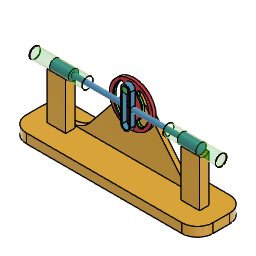
ScotchYoke (Autodesk Fusion 360 design; units mm, degrees)
Autodesk Fusion 360 part; units mm, degrees
sketch "BaseSketch" plane through (0, 0, 0) normal (0, 0, 1) x (1, 0, 0) in component "Holder"
  line L0 (30, 4.8) -> (30, 7.5)
  line L1 (27.5, 10) -> (2.5, 10)
  line L2 (0, 7.5) -> (0, 4.8)
  arc A0 (2.5, 10) -> (0, 7.5) centre (2.5, 7.5) ccw
  arc A1 (30, 7.5) -> (27.5, 10) centre (27.5, 7.5) ccw
  line L3 (15, 0) -> (15, 10) construction
  line L4 (2.75, 6.5) -> (2.75, 5.8)
  line L5 (5.75, 6.15) -> (5.75, 6.9)
  line L6 (5.75, 6.9) -> (2.75, 6.9)
  line L7 (2.75, 6.9) -> (2.75, 5.4)
  line L8 (2.75, 5.4) -> (5.75, 5.4)
  line L9 (5.75, 5.4) -> (5.75, 6.9)
  line L10 (5.75, 2.3) -> (2.5, 2.3)
  line L11 (0, 2.3) -> (0, 2.5)
  line L12 (5.75, 2.3) -> (27.5, 2.3)
  arc A2 (0, 4.8) -> (2.5, 2.3) centre (2.5, 4.8) ccw
  arc A3 (27.5, 2.3) -> (30, 4.8) centre (27.5, 4.8) ccw
  line L13 (27.25, 6.9) -> (27.25, 5.4)
  line L14 (24.25, 6.9) -> (27.25, 6.9)
  line L15 (24.25, 5.4) -> (24.25, 6.9)
  line L16 (27.25, 5.4) -> (24.25, 5.4)
  point P0 (30, 0)
  point P1 (0, 10)
  point P2 (27.5, 7.5)
  dimension "d1" = 30
  dimension "d3" = 2.5
  dimension "d4" = 2.5
  dimension "d81" = 3
  dimension "d82" = 1.5
  dimension "d83" = 3.1
  dimension "d84" = 2.5
  dimension "d85" = 2.5
  constraint vertical L0
  constraint horizontal L1
  constraint vertical L2
  constraint coincident P1 L1
  constraint coincident P1 L2
  constraint tangent L1 A0
  constraint tangent L2 A0
  constraint tangent L0 A1
  constraint tangent L1 A1
  constraint coincident P0 L0
  constraint coincident origin L2
  constraint midpoint L1 L3.end
  constraint vertical L4
  constraint horizontal L6
  constraint vertical L7
  constraint horizontal L8
  constraint vertical L9
  constraint perpendicular L10 L11
  constraint perpendicular L0 L12
  constraint coincident L11.start L10
  constraint coincident L2 L11.end
  constraint tangent L10 A2
  constraint tangent L2 A2
  constraint tangent L12 A3
  constraint tangent L0 A3
  constraint symmetric A0.centre L3 P2
  constraint symmetric L3 L5.end L14.start
  constraint symmetric L3 L6.end L13.start
  constraint symmetric L3 L7.end L13.end
  constraint symmetric L3 L8.end L15.start
  measures "d1" distance of origin P0
  measures "d3" radius of A0
  measures "d4" radius of A1
  measures "d81" distance of L5.end L6.end
  measures "d82" distance of L5.end L8.end
  measures "d83" distance of L8.end L10.start
  measures "d84" radius of A2
  measures "d85" radius of A3
extrude "Extrude1" add sketch "BaseSketch" along normal blind 1.5 contours L0 L1 L2 A0 A1 L10 L12 A2 A3 | L4 L5 L6 L7 L8 L9 | L13 L14 L15 L16 makes body 1 in component "Holder"
sketch "CrankSupportSketch" plane through (0, 0, 0) normal (0, 1, 0) x (1, 0, 0) in component "Holder"
  line L0 (13.2512, -9.8397) -> (6.5, -1.5)
  line L1 (6.5, -1.5) -> (15, -1.5)
  line L2 (16.7488, -9.8397) -> (23.5, -1.5)
  line L3 (23.5, -1.5) -> (15, -1.5)
  arc A0 (13.2512, -9.8397) -> (16.7488, -9.8397) centre (15, -8.424) ccw
  circle A1 centre (15, -9.5) radius 0.5
  line L4 (15, -9.5) -> (2.1474, -9.5)
  dimension "d12" = 2.25
  dimension "d13" = 1
  constraint horizontal L1
  constraint tangent L0 A0
  constraint tangent L2 A0
  constraint coincident A1.centre L4.start
  constraint horizontal L4
  measures "d12" radius of A0
  measures "d13" diameter of A1
extrude "Extrude3" add sketch "CrankSupportSketch" against normal blind 0.75 from surface at 8 contours L0 L1 L2 L3 A0 | A1 bodies 1 in component "Holder"
extrude "Extrude4" cut sketch "CrankSupportSketch" along normal blind 7.75 contours A1 bodies 1 in component "Holder"
move_face "OffsetFaces1" offset -0.05 1 faces at (15.3986, 7.4167, 9.1981) on bodies 1 in component "Holder"
fillet "Fillet1" radius 4.25 1 edges at (23.5, 7.625, 1.5) on bodies 1 in component "Holder"
fillet "Fillet2" radius 4.25 1 edges at (6.5, 7.625, 1.5) on bodies 1 in component "Holder"
sketch "CrankSketch" plane through (0, 7.75, 0) normal (0, -1, 0) x (1, 0, 0) in component "Crank"
  circle A0 centre (15, 9.5) radius 0.55
  circle A1 centre (15, 9.5) radius 3.5
  circle A2 centre (15, 9.5) radius 0.55
  circle A3 centre (15, 9.5) radius 0.5
  circle A4 centre (15, 12) radius 0.5
  line L0 (13.5, 7.5) -> (14, 7.5) construction
  line L1 (13.5, 11.5) -> (14, 11.5) construction
  arc A5 (13.8536, 11.1464) -> (13.1464, 11.8536) centre (13.5, 11.5) ccw
  arc A6 (13.1464, 7.1464) -> (13.8536, 7.8536) centre (13.5, 7.5) ccw
  arc A7 (13.1464, 11.8536) -> (13.1464, 7.1464) centre (15.5, 9.5) ccw
  arc A8 (13.8536, 11.1464) -> (13.8536, 7.8536) centre (15.5, 9.5) ccw
  arc A9 (16.1005, 7.8536) -> (16.1005, 11.1464) centre (14.454, 9.5) ccw
  arc A10 (16.8076, 11.8536) -> (16.1005, 11.1464) centre (16.454, 11.5) ccw
  arc A11 (16.8076, 7.1464) -> (16.8076, 11.8536) centre (14.454, 9.5) ccw
  arc A12 (16.1005, 7.8536) -> (16.8076, 7.1464) centre (16.454, 7.5) ccw
  dimension "d34" = 1
  constraint concentric A0 A1
  constraint concentric A0 A2
  constraint concentric A1 A3
  constraint horizontal L0
  constraint coincident L0.start A6.centre
  constraint horizontal L1
  constraint coincident L1.start A5.centre
  constraint tangent A6 A7
  constraint tangent A6 A8
  measures "d34" diameter of A3
extrude "Extrude1'" add sketch "CrankSketch" along normal blind 0.5 from surface at 0.6 separate body contours A0 A2 | A1 makes body 2 in component "Crank"
extrude "Extrude2" add sketch "CrankSketch" along normal blind 1.5 from surface at 0.6 contours A4 bodies 2 in component "Crank"
extrude "Extrude3'" add sketch "CrankSketch" along normal blind 1.2 from surface at 0.05 contours A3 bodies 2 in component "Crank"
sketch "SliderSketch" plane through (0, 6.65, 0) normal (0, -1, 0) x (1, 0, 0) in component "Slider&Piston"
  arc A0 (13.1464, 11.8536) -> (13.1464, 7.1464) centre (15.5, 9.5) ccw
  arc A1 (13.8536, 11.1464) -> (13.1464, 11.8536) centre (13.5, 11.5) ccw
  arc A2 (13.8536, 11.1464) -> (13.8536, 7.8536) centre (15.5, 9.5) ccw
  arc A3 (13.1464, 7.1464) -> (13.8536, 7.8536) centre (13.5, 7.5) ccw
  arc A4 (16.1005, 7.8536) -> (16.8076, 7.1464) centre (16.454, 7.5) ccw
  arc A5 (16.1005, 7.8536) -> (16.1005, 11.1464) centre (14.454, 9.5) ccw
  arc A6 (16.8076, 11.8536) -> (16.1005, 11.1464) centre (16.454, 11.5) ccw
  arc A7 (16.8076, 7.1464) -> (16.8076, 11.8536) centre (14.454, 9.5) ccw
  circle A8 centre (15, 12) radius 0.5
  circle A9 centre (15, 9.5) radius 3.5
  arc A10 (15.55, 12.0055) -> (14.45, 12.0055) centre (15, 12) ccw
  arc A11 (15.75, 12.0075) -> (14.25, 12.0075) centre (15, 12) ccw
  line L0 (14.45, 12.0055) -> (14.45, 9.5055)
  line L1 (14.25, 12.0075) -> (14.25, 9.5075)
  line L2 (14.25, 9.5075) -> (15.8, 9.5075) construction
  line L3 (15, 12) -> (15, 9.5) construction
  line L4 (15.55, 12.0055) -> (15.55, 9.5055)
  line L5 (15.75, 12.0075) -> (15.75, 9.5075)
  arc A12 (14.45, 7.0095) -> (15.55, 7.0095) centre (15, 7.015) ccw
  line L6 (14.45, 7.0095) -> (14.45, 9.5095)
  line L7 (15.55, 7.0095) -> (15.55, 9.5095)
  line L8 (15.75, 7.0075) -> (15.75, 9.5075)
  arc A13 (14.25, 7.0075) -> (15.75, 7.0075) centre (15, 7.015) ccw
  line L9 (14.25, 7.0075) -> (14.25, 9.5075)
  circle A14 centre (15, 9.5) radius 0.5
  dimension "d61" = 1.1
  dimension "d62" = 0.2
  dimension "d64" = 2.5
  constraint concentric A8 A10
  constraint vertical L0
  constraint vertical L1
  constraint perpendicular L1 L2
  constraint coincident A8.centre A10.centre
  constraint coincident A9.centre L3.end
  constraint symmetric A10.end L3 A10.start
  constraint symmetric A11.end L3 A11.start
  constraint symmetric L0.end L3 L4.end
  constraint symmetric L1.end L3 L5.end
  constraint symmetric A10.end L2 A12.start
  constraint symmetric A10.start L2 A12.end
  constraint symmetric A10 L2 A12
  constraint symmetric A11.end L2 A13.start
  constraint symmetric A11.start L2 L8.start
  constraint symmetric A11 L2 A13
  constraint symmetric L0.end L2 L6.end
  constraint symmetric L1.end L2 L9.end
  constraint symmetric L2 A10.start A12.end
  constraint symmetric L2 L4.end L7.end
  constraint symmetric L2 A11.start L8.start
  constraint symmetric L2 L5.end L8.end
  measures "d61" diameter of A10
  measures "d64" distance of A10.end L0.end
extrude "Extrude1''" add sketch "SliderSketch" along normal blind 0.8 from surface at 0.1 separate body contours A11 L1 L5 L8 A13 L9 makes body 3 in component "Slider&Piston"
sketch "PistonSketch" plane through (14.25, 0, 0) normal (-1, 0, 0) x (0, -1, 0) in component "Slider&Piston"
  line L0 (-6.55, 12.0075) -> (-6.55, 7.0075)
  line L1 (-6.55, 7.0075) -> (-5.75, 7.0075)
  line L2 (-5.75, 7.0075) -> (-5.75, 12.0075)
  line L3 (-5.75, 12.0075) -> (-6.55, 12.0075)
  circle A0 centre (-6.15, 9.5075) radius 0.375
  circle A1 centre (-6.15, 9.5075) radius 0.825
  circle A2 centre (-6.15, 9.5075) radius 0.85
  dimension "d69" = 0.75
  dimension "d119" = 1.65
  dimension "d136" = 1.7
  constraint concentric A0 A1
  constraint concentric A0 A2
  measures "d69" diameter of A0
  measures "d119" diameter of A1
  measures "d136" diameter of A2
extrude "Extrude2'" add sketch "PistonSketch" along normal blind 8 contours A0 bodies 3 in component "Slider&Piston"
extrude "Extrude3''" add sketch "PistonSketch" against normal blind 8 from surface at -1.49 contours A0 bodies 3 in component "Slider&Piston"
extrude "Extrude9" add sketch "BaseSketch" along normal blind 8 from surface at 1.5 contours L4 L5 L6 L7 L8 L9 | L13 L14 L15 L16 bodies 1 in component "Holder"
sketch "CylinderCutSketch" plane through (6.25, 0, 0) normal (-1, 0, 0) x (0, -1, 0) in component "Holder"
  circle A0 centre (-6.15, 9.5075) radius 0.375
  circle A1 centre (-6.15, 9.5075) radius 0.9
extrude "Extrude11" cut sketch "CylinderCutSketch" along normal mid plane 43 contours A0 | A1 bodies 1 in component "Holder"
sketch "PistonLeftSketch" plane through (6.25, 0, 0) normal (-1, 0, 0) x (0, -1, 0) in component "PistonSupports"
  circle A0 centre (-6.15, 9.5075) radius 0.375
  circle A1 centre (-6.15, 9.5075) radius 0.85
  circle A2 centre (-6.15, 9.5075) radius 0.9
  dimension "d100" = 1.7
  dimension "d102" = 0.05
  measures "d100" diameter of A1
sketch "PistonRightSketch" plane through (23.74, 0, 0) normal (1, 0, 0) x (0, 1, 0) in component "PistonSupports"
  circle A0 centre (6.15, 9.5075) radius 0.375
  circle A1 centre (6.15, 9.5075) radius 0.9
  circle A2 centre (6.15, 9.5075) radius 0.85
  dimension "d103" = 1.8
  dimension "d104" = -0.05
  constraint concentric A0 A1
  measures "d103" diameter of A1
extrude "Extrude5" add sketch "PistonLeftSketch" along normal blind 6.25 and the other way blind 2.25 separate body contours A2 makes body 4 in component "PistonSupports"
extrude "Extrude6" add sketch "PistonLeftSketch" along normal blind 0.1 from surface at 6.15 contours A0 | A1 bodies 4 in component "PistonSupports"
extrude "Extrude7" add sketch "PistonRightSketch" along normal blind 6.25 and the other way blind 2.25 separate body contours A1 makes body 5 in component "PistonSupports"
extrude "Extrude8" add sketch "PistonRightSketch" along normal blind 0.1 from surface at 6.15 contours A0 | A2 bodies 5 in component "PistonSupports"
extrude "Extrude4'" add sketch "PistonSketch" along normal blind 3 from surface at 8 contours L0 L2 A1 | L0 A1 | L2 A1 | A0 bodies 3 in component "Slider&Piston"
extrude "Extrude5'" add sketch "PistonSketch" against normal blind 3 from surface at -9.49 contours L0 L2 A1 | L0 A1 | L2 A1 | A0 bodies 3 in component "Slider&Piston"
fillet "Fillet1'" radius 0.1 16 edges at (13.1716, 7.15, 9.5) (13.8536, 7.15, 7.1464) (12.1716, 7.15, 9.5) (13.8536, 7.15, 11.8536) (12.1716, 6.65, 9.5) (13.8536, 6.65, 11.8536) (13.1716, 6.65, 9.5) (13.8536, 6.65, 7.1464) (17.7825, 6.65, 9.5) (16.1005, 6.65, 7.1464) (16.7825, 6.65, 9.5) (16.1005, 6.65, 11.8536) (17.7825, 7.15, 9.5) (16.1005, 7.15, 7.1464) (16.7825, 7.15, 9.5) (16.1005, 7.15, 11.8536) on bodies 2 in component "Crank"
component "Holder" placed x (1, 0, 0) y (0, 1, 0) z (0, 0, 1) at (0, 0, 0)
component "Crank" placed x (1, 0, 0) y (0, 1, 0) z (0, 0, 1) at (0, 0, 0)
component "Slider&Piston" placed x (1, 0, 0) y (0, 1, 0) z (0, 0, 1) at (0, 0, 0)
component "PistonSupports" placed x (1, 0, 0) y (0, 1, 0) z (0, 0, 1) at (0, 0, 0)
named bodies: "HolderBody", "CrankBody.", "Slider&Piston", "PistonLeftSupport", "PistonRightSupport"
